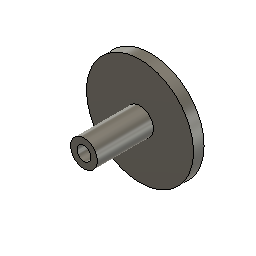
rueda_scotch (Autodesk Fusion 360 design; units mm, degrees)
part number: 2026-04-14-10-55-13-191
Autodesk Fusion 360 part; units mm, degrees
sketch "Boceto1" plane through (0, 0, 0) normal (0, 0, 1) x (1, 0, 0)
  circle A0 centre (0, 0) radius 20
  circle A1 centre (0, 0) radius 2.6
  circle A2 centre (-7.8095, 9.1111) radius 3
  dimension "d1" = 40
  dimension "d2" = 5.2
  dimension "d20" = 6
  dimension "d21" = 12
  constraint coincident A0.centre A1.centre
  constraint concentric A0 A1
  measures "d1" diameter of A0
  measures "d2" diameter of A1
  measures "d20" diameter of A2
  measures "d21" distance of A0.centre A2.centre
extrude "Extruir1" add sketch "Boceto1" along normal blind 4 contours A0 | A1 | A2
sketch "Boceto2" plane through (0, 0, 4) normal (0, 0, 1) x (1, 0, 0)
  circle A0 centre (0, 0) radius 20
  circle A1 centre (0, 0) radius 2.6
  circle A2 centre (0, 0) radius 5
  dimension "d14" = 5.2
  dimension "d15" = 10
  constraint coincident A0.centre A1.centre
  measures "d14" diameter of A1
  measures "d15" diameter of A2
extrude "Extruir2" add sketch "Boceto2" along normal blind 21 contours A2
sketch "Boceto3" plane through (0, 0, 0) normal (1, 0, 0) x (0, 0, -1)
  circle A0 centre (-22, 0) radius 1
  dimension "d18" = 2
  measures "d18" diameter of A0
extrude "Extruir4" add sketch "Boceto1" against normal blind 8 contours A2
fillet "Empalme1" radius 1 1 edges at (-10.6065, 10.1959, -8)
